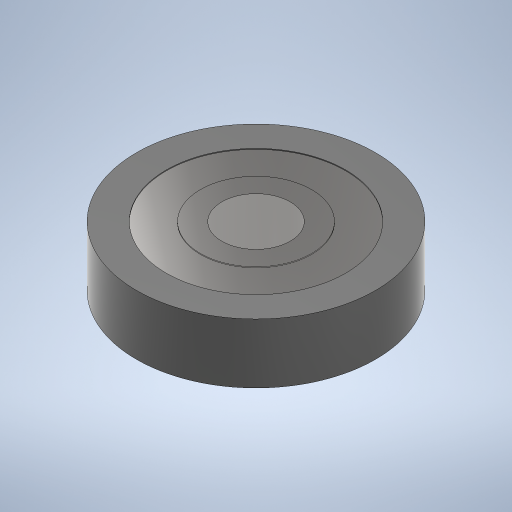
# Autodesk Inventor part: Gbear_28_8
Saved by Autodesk Inventor 2024.2 (Build 282272000, 272)
## iProperties
Created: 2024-03-24
Part Number: Gbear_28_8
Material: ステンレス鋼
Document SubType Name: Modeling
Designer: fhbdh
Density: 8 g/cm^3
Appearance: 半つや出し
Author: fhbdh
Autodesk Inventor part; units mm, degrees
ref_plane "YZ Plane" through (0, 0, 0) normal (1, 0, 0) x (0, 1, 0)
ref_plane "XZ Plane" through (0, 0, 0) normal (0, 1, 0) x (-1, 0, 0)
ref_plane "XY Plane" through (0, 0, 0) normal (0, 0, 1) x (1, 0, 0)
sketch "スケッチ1" plane through (0, 0, 0) normal (0, 0, 1) x (1, 0, 0)
  line L0 (-14, 3.5) -> (-14, -3.5)
  line L1 (-14, -3.5) -> (-10.5, -3.5)
  line L2 (-10.5, -3.5) -> (-10.5, -3.4)
  line L3 (-10.5, -3.4) -> (-6.5, -3.4)
  line L4 (-6.5, -3.4) -> (-6.5, -3.5)
  line L5 (-6.5, -3.5) -> (-4, -3.5)
  line L6 (-4, -3.5) -> (-4, 3.5)
  line L7 (0, 0) -> (-14, 0) construction
  line L8 (0, 0) -> (0, 3.5) construction
  line L9 (-14, 3.5) -> (-10.5, 3.5)
  line L10 (-10.5, 3.5) -> (-10.5, 3.4)
  line L11 (-10.5, 3.4) -> (-6.5, 3.4)
  line L12 (-6.5, 3.4) -> (-6.5, 3.5)
  line L13 (-6.5, 3.5) -> (-4, 3.5)
  dimension "d0" = 0.1
  dimension "d1" = 7
  dimension "d2" = 4
  dimension "d3" = 14
  dimension "d4" = 3.5
  dimension "d5" = 2.5
  constraints: 28 end point, 5 perpendicular, 5 point on line, 5 symmetric about line, 2 vertical, 1 horizontal, 1 midpoint
  measures "d0" distance of L3.end L4.end
  measures "d1" distance of L0.start L0.end
  measures "d2" distance from line of L7.start L6
  measures "d3" distance between parallel lines of L0 L8
  measures "d4" distance of L0.end L1.end
  measures "d5" distance of L4.end L5.end
revolve "回転1" add sketch "スケッチ1" angle 360 about axis through (0, 0, 0) along (0, 1, 0)
